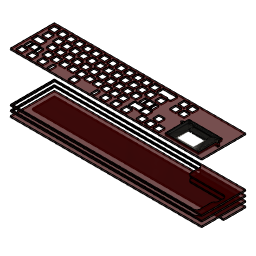
Snack  Case Concept V1 v1 (Autodesk Fusion 360 design; units mm, degrees)
Autodesk Fusion 360 part; units mm, degrees
(part 1 of 3)
sketch "plate-20210524-013526" plane through (0, 0, 0) normal (0, 0, 1) x (1, 0, 0)
  line L0 (286.3938, -78.725) -> (299.3938, -78.725)
  arc A0 (285.8938, -92.225) -> (286.3938, -92.725) centre (286.3938, -92.225) ccw
  arc A1 (299.3938, -92.725) -> (299.8938, -92.225) centre (299.3938, -92.225) ccw
  arc A2 (373.7125, -79.225) -> (373.2125, -78.725) centre (373.2125, -79.225) ccw
  arc A3 (359.7125, -92.225) -> (360.2125, -92.725) centre (360.2125, -92.225) ccw
  arc A4 (276.0813, -79.225) -> (275.5813, -78.725) centre (275.5813, -79.225) ccw
  arc A5 (354.6625, -79.225) -> (354.1625, -78.725) centre (354.1625, -79.225) ccw
  arc A6 (354.1625, -92.725) -> (354.6625, -92.225) centre (354.1625, -92.225) ccw
  line L1 (341.1625, -78.725) -> (354.1625, -78.725)
  arc A7 (335.1125, -92.725) -> (335.6125, -92.225) centre (335.1125, -92.225) ccw
  arc A8 (335.6125, -79.225) -> (335.1125, -78.725) centre (335.1125, -79.225) ccw
  arc A9 (340.6625, -92.225) -> (341.1625, -92.725) centre (341.1625, -92.225) ccw
  line L2 (360.2125, -92.725) -> (373.2125, -92.725)
  line L3 (373.7125, -79.225) -> (373.7125, -92.225)
  line L4 (299.8938, -79.225) -> (299.8938, -92.225)
  line L5 (322.1125, -78.725) -> (335.1125, -78.725)
  arc A10 (321.6125, -92.225) -> (322.1125, -92.725) centre (322.1125, -92.225) ccw
  line L6 (354.6625, -79.225) -> (354.6625, -92.225)
  line L7 (285.8938, -79.225) -> (285.8938, -92.225)
  line L8 (359.7125, -79.225) -> (359.7125, -92.225)
  line L9 (322.1125, -92.725) -> (335.1125, -92.725)
  line L10 (286.3938, -92.725) -> (299.3938, -92.725)
  line L11 (341.1625, -92.725) -> (354.1625, -92.725)
  line L12 (360.2125, -78.725) -> (373.2125, -78.725)
  arc A11 (322.1125, -78.725) -> (321.6125, -79.225) centre (322.1125, -79.225) ccw
  arc A12 (341.1625, -78.725) -> (340.6625, -79.225) centre (341.1625, -79.225) ccw
  line L13 (335.6125, -79.225) -> (335.6125, -92.225)
  arc A13 (286.3938, -78.725) -> (285.8938, -79.225) centre (286.3938, -79.225) ccw
  arc A14 (275.5813, -92.725) -> (276.0813, -92.225) centre (275.5813, -92.225) ccw
  arc A15 (360.2125, -78.725) -> (359.7125, -79.225) centre (360.2125, -79.225) ccw
  arc A16 (45.3875, -16.025) -> (45.8875, -16.525) centre (45.8875, -16.025) ccw
  arc A17 (299.8938, -79.225) -> (299.3938, -78.725) centre (299.3938, -79.225) ccw
  arc A18 (262.0813, -92.225) -> (262.5813, -92.725) centre (262.5813, -92.225) ccw
  line L14 (321.6125, -79.225) -> (321.6125, -92.225)
  line L15 (340.6625, -79.225) -> (340.6625, -92.225)
  arc A19 (373.2125, -92.725) -> (373.7125, -92.225) centre (373.2125, -92.225) ccw
  line L16 (64.4375, -3.025) -> (64.4375, -16.025)
  line L17 (160.1875, -2.525) -> (173.1875, -2.525)
  line L18 (135.5875, -3.025) -> (135.5875, -16.025)
  arc A20 (116.5375, -3.025) -> (116.0375, -2.525) centre (116.0375, -3.025) ccw
  arc A21 (58.8875, -16.525) -> (59.3875, -16.025) centre (58.8875, -16.025) ccw
  arc A22 (160.1875, -2.525) -> (159.6875, -3.025) centre (160.1875, -3.025) ccw
  arc A23 (173.1875, -16.525) -> (173.6875, -16.025) centre (173.1875, -16.025) ccw
  arc A24 (97.4875, -3.025) -> (96.9875, -2.525) centre (96.9875, -3.025) ccw
  line L19 (140.6375, -3.025) -> (140.6375, -16.025)
  line L20 (178.7375, -3.025) -> (178.7375, -16.025)
  arc A25 (83.4875, -16.025) -> (83.9875, -16.525) centre (83.9875, -16.025) ccw
  line L21 (160.1875, -16.525) -> (173.1875, -16.525)
  arc A26 (159.6875, -16.025) -> (160.1875, -16.525) centre (160.1875, -16.025) ccw
  arc A27 (64.4375, -16.025) -> (64.9375, -16.525) centre (64.9375, -16.025) ccw
  arc A28 (45.8875, -2.525) -> (45.3875, -3.025) centre (45.8875, -3.025) ccw
  arc A29 (102.5375, -16.025) -> (103.0375, -16.525) centre (103.0375, -16.025) ccw
  line L22 (78.4375, -3.025) -> (78.4375, -16.025)
  arc A30 (154.6375, -3.025) -> (154.1375, -2.525) centre (154.1375, -3.025) ccw
  arc A31 (135.0875, -16.525) -> (135.5875, -16.025) centre (135.0875, -16.025) ccw
  line L23 (64.9375, -2.525) -> (77.9375, -2.525)
  line L24 (141.1375, -2.525) -> (154.1375, -2.525)
  line L25 (121.5875, -3.025) -> (121.5875, -16.025)
  line L26 (154.6375, -3.025) -> (154.6375, -16.025)
  line L27 (102.5375, -3.025) -> (102.5375, -16.025)
  line L28 (159.6875, -3.025) -> (159.6875, -16.025)
  line L29 (45.3875, -3.025) -> (45.3875, -16.025)
  line L30 (122.0875, -2.525) -> (135.0875, -2.525)
  arc A32 (116.0375, -16.525) -> (116.5375, -16.025) centre (116.0375, -16.025) ccw
  line L31 (103.0375, -2.525) -> (116.0375, -2.525)
  line L32 (179.2375, -16.525) -> (192.2375, -16.525)
  line L33 (83.4875, -3.025) -> (83.4875, -16.025)
  line L34 (116.5375, -3.025) -> (116.5375, -16.025)
  line L35 (103.0375, -16.525) -> (116.0375, -16.525)
  line L36 (97.4875, -3.025) -> (97.4875, -16.025)
  arc A33 (59.3875, -3.025) -> (58.8875, -2.525) centre (58.8875, -3.025) ccw
  line L37 (192.7375, -3.025) -> (192.7375, -16.025)
  arc A34 (141.1375, -2.525) -> (140.6375, -3.025) centre (141.1375, -3.025) ccw
  arc A35 (64.9375, -2.525) -> (64.4375, -3.025) centre (64.9375, -3.025) ccw
  arc A36 (77.9375, -16.525) -> (78.4375, -16.025) centre (77.9375, -16.025) ccw
  arc A37 (135.5875, -3.025) -> (135.0875, -2.525) centre (135.0875, -3.025) ccw
  line L38 (64.9375, -16.525) -> (77.9375, -16.525)
  arc A38 (122.0875, -2.525) -> (121.5875, -3.025) centre (122.0875, -3.025) ccw
  arc A39 (268.9375, -3.025) -> (268.4375, -2.525) centre (268.4375, -3.025) ccw
  arc A40 (198.2875, -2.525) -> (197.7875, -3.025) centre (198.2875, -3.025) ccw
  line L39 (235.8875, -3.025) -> (235.8875, -16.025)
  line L40 (236.3875, -2.525) -> (249.3875, -2.525)
  arc A41 (287.9875, -3.025) -> (287.4875, -2.525) centre (287.4875, -3.025) ccw
  arc A42 (274.4875, -2.525) -> (273.9875, -3.025) centre (274.4875, -3.025) ccw
  arc A43 (236.3875, -2.525) -> (235.8875, -3.025) centre (236.3875, -3.025) ccw
  line L41 (294.1245, -17.025) -> (294.1245, -18.025)
  arc A44 (121.5875, -16.025) -> (122.0875, -16.525) centre (122.0875, -16.025) ccw
  arc A45 (83.9875, -2.525) -> (83.4875, -3.025) centre (83.9875, -3.025) ccw
  line L42 (83.9875, -16.525) -> (96.9875, -16.525)
  line L43 (122.0875, -16.525) -> (135.0875, -16.525)
  line L44 (198.2875, -2.525) -> (211.2875, -2.525)
  line L45 (83.9875, -2.525) -> (96.9875, -2.525)
  arc A46 (324.5005, -18.525) -> (325.0005, -18.025) centre (324.5005, -18.025) ccw
  line L46 (294.6245, -18.525) -> (300.6245, -18.525)
  arc A47 (178.7375, -16.025) -> (179.2375, -16.525) centre (179.2375, -16.025) ccw
  line L47 (301.1245, -17.025) -> (301.1245, -18.025)
  line L48 (254.9375, -3.025) -> (254.9375, -16.025)
  arc A48 (230.8375, -3.025) -> (230.3375, -2.525) centre (230.3375, -3.025) ccw
  line L49 (230.8375, -3.025) -> (230.8375, -16.025)
  line L50 (45.8875, -2.525) -> (58.8875, -2.525)
  line L51 (273.9875, -3.025) -> (273.9875, -16.025)
  line L52 (141.1375, -16.525) -> (154.1375, -16.525)
  line L53 (197.7875, -3.025) -> (197.7875, -16.025)
  arc A49 (249.8875, -3.025) -> (249.3875, -2.525) centre (249.3875, -3.025) ccw
  line L54 (216.8375, -3.025) -> (216.8375, -16.025)
  line L55 (249.8875, -3.025) -> (249.8875, -16.025)
  arc A50 (217.3375, -2.525) -> (216.8375, -3.025) centre (217.3375, -3.025) ccw
  arc A51 (216.8375, -16.025) -> (217.3375, -16.525) centre (217.3375, -16.025) ccw
  line L56 (268.9375, -3.025) -> (268.9375, -16.025)
  line L57 (45.8875, -16.525) -> (58.8875, -16.525)
  arc A52 (140.6375, -16.025) -> (141.1375, -16.525) centre (141.1375, -16.025) ccw
  line L58 (179.2375, -2.525) -> (192.2375, -2.525)
  line L59 (217.3375, -16.525) -> (230.3375, -16.525)
  arc A53 (197.7875, -16.025) -> (198.2875, -16.525) centre (198.2875, -16.025) ccw
  arc A54 (273.9875, -16.025) -> (274.4875, -16.525) centre (274.4875, -16.025) ccw
  arc A55 (96.9875, -16.525) -> (97.4875, -16.025) centre (96.9875, -16.025) ccw
  line L60 (236.3875, -16.525) -> (249.3875, -16.525)
  line L61 (59.3875, -3.025) -> (59.3875, -16.025)
  line L62 (303.0625, -2.525) -> (316.0625, -2.525)
  arc A56 (235.8875, -16.025) -> (236.3875, -16.525) centre (236.3875, -16.025) ccw
  arc A57 (268.4375, -16.525) -> (268.9375, -16.025) centre (268.4375, -16.025) ccw
  arc A58 (211.2875, -16.525) -> (211.7875, -16.025) centre (211.2875, -16.025) ccw
  line L63 (173.6875, -3.025) -> (173.6875, -16.025)
  line L64 (318.5005, -18.525) -> (324.5005, -18.525)
  line L65 (211.7875, -3.025) -> (211.7875, -16.025)
  arc A59 (78.4375, -3.025) -> (77.9375, -2.525) centre (77.9375, -3.025) ccw
  arc A60 (103.0375, -2.525) -> (102.5375, -3.025) centre (103.0375, -3.025) ccw
  arc A61 (255.4375, -2.525) -> (254.9375, -3.025) centre (255.4375, -3.025) ccw
  line L66 (255.4375, -2.525) -> (268.4375, -2.525)
  arc A62 (154.1375, -16.525) -> (154.6375, -16.025) centre (154.1375, -16.025) ccw
  arc A63 (173.6875, -3.025) -> (173.1875, -2.525) centre (173.1875, -3.025) ccw
  arc A64 (192.7375, -3.025) -> (192.2375, -2.525) centre (192.2375, -3.025) ccw
  arc A65 (179.2375, -2.525) -> (178.7375, -3.025) centre (179.2375, -3.025) ccw
  arc A66 (211.7875, -3.025) -> (211.2875, -2.525) centre (211.2875, -3.025) ccw
  line L67 (255.4375, -16.525) -> (268.4375, -16.525)
  line L68 (274.4875, -16.525) -> (287.4875, -16.525)
  line L69 (131.1125, -22.075) -> (131.1125, -35.075)
  line L70 (74.4625, -21.575) -> (87.4625, -21.575)
  line L71 (287.9875, -3.025) -> (287.9875, -16.025)
  arc A67 (287.4875, -16.525) -> (287.9875, -16.025) centre (287.4875, -16.025) ccw
  arc A68 (318.0005, -18.025) -> (318.5005, -18.525) centre (318.5005, -18.025) ccw
  arc A69 (64.15, -22.075) -> (63.65, -21.575) centre (63.65, -22.075) ccw
  arc A70 (126.0625, -22.075) -> (125.5625, -21.575) centre (125.5625, -22.075) ccw
  line L72 (131.6125, -35.575) -> (144.6125, -35.575)
  line L73 (50.65, -35.575) -> (63.65, -35.575)
  line L74 (73.9625, -22.075) -> (73.9625, -35.075)
  arc A71 (373.2125, -16.525) -> (373.7125, -16.025) centre (373.2125, -16.025) ccw
  arc A72 (300.6245, -18.525) -> (301.1245, -18.025) centre (300.6245, -18.025) ccw
  line L75 (217.3375, -2.525) -> (230.3375, -2.525)
  arc A73 (144.6125, -35.575) -> (145.1125, -35.075) centre (144.6125, -35.075) ccw
  arc A74 (192.2375, -16.525) -> (192.7375, -16.025) centre (192.2375, -16.025) ccw
  line L76 (126.0625, -22.075) -> (126.0625, -35.075)
  arc A75 (50.65, -21.575) -> (50.15, -22.075) centre (50.65, -22.075) ccw
  line L77 (150.6625, -35.575) -> (163.6625, -35.575)
  arc A76 (93.5125, -21.575) -> (93.0125, -22.075) centre (93.5125, -22.075) ccw
  arc A77 (230.3375, -16.525) -> (230.8375, -16.025) centre (230.3375, -16.025) ccw
  line L78 (198.2875, -16.525) -> (211.2875, -16.525)
  arc A78 (87.9625, -22.075) -> (87.4625, -21.575) centre (87.4625, -22.075) ccw
  line L79 (107.0125, -22.075) -> (107.0125, -35.075)
  line L80 (373.7125, -3.025) -> (373.7125, -16.025)
  line L81 (150.1625, -22.075) -> (150.1625, -35.075)
  arc A79 (254.9375, -16.025) -> (255.4375, -16.525) centre (255.4375, -16.025) ccw
  arc A80 (360.2125, -2.525) -> (359.7125, -3.025) centre (360.2125, -3.025) ccw
  line L82 (325.0005, -17.025) -> (325.0005, -18.025)
  line L83 (354.6625, -3.025) -> (354.6625, -16.025)
  arc A81 (145.1125, -22.075) -> (144.6125, -21.575) centre (144.6125, -22.075) ccw
  line L84 (164.1625, -22.075) -> (164.1625, -35.075)
  line L85 (341.1625, -16.525) -> (354.1625, -16.525)
  arc A82 (107.0125, -22.075) -> (106.5125, -21.575) centre (106.5125, -22.075) ccw
  arc A83 (87.4625, -35.575) -> (87.9625, -35.075) centre (87.4625, -35.075) ccw
  line L86 (93.5125, -35.575) -> (106.5125, -35.575)
  arc A84 (73.9625, -35.075) -> (74.4625, -35.575) centre (74.4625, -35.075) ccw
  arc A85 (354.1625, -16.525) -> (354.6625, -16.025) centre (354.1625, -16.025) ccw
  line L87 (93.0125, -22.075) -> (93.0125, -35.075)
  line L88 (274.4875, -2.525) -> (287.4875, -2.525)
  arc A86 (373.7125, -3.025) -> (373.2125, -2.525) centre (373.2125, -3.025) ccw
  arc A87 (50.15, -35.075) -> (50.65, -35.575) centre (50.65, -35.075) ccw
  line L89 (112.5625, -21.575) -> (125.5625, -21.575)
  line L90 (360.2125, -2.525) -> (373.2125, -2.525)
  arc A88 (93.0125, -35.075) -> (93.5125, -35.575) centre (93.5125, -35.075) ccw
  line L91 (150.6625, -21.575) -> (163.6625, -21.575)
  arc A89 (74.4625, -21.575) -> (73.9625, -22.075) centre (74.4625, -22.075) ccw
  line L92 (360.2125, -16.525) -> (373.2125, -16.525)
  line L93 (64.15, -22.075) -> (64.15, -35.075)
  arc A90 (112.0625, -35.075) -> (112.5625, -35.575) centre (112.5625, -35.075) ccw
  arc A91 (340.6625, -16.025) -> (341.1625, -16.525) centre (341.1625, -16.025) ccw
  arc A92 (249.3875, -16.525) -> (249.8875, -16.025) centre (249.3875, -16.025) ccw
  line L94 (145.1125, -22.075) -> (145.1125, -35.075)
  line L95 (318.0005, -17.025) -> (318.0005, -18.025)
  arc A93 (125.5625, -35.575) -> (126.0625, -35.075) centre (125.5625, -35.075) ccw
  line L96 (303.0625, -16.525) -> (316.0625, -16.525)
  arc A94 (354.6625, -3.025) -> (354.1625, -2.525) centre (354.1625, -3.025) ccw
  line L97 (87.9625, -22.075) -> (87.9625, -35.075)
  arc A95 (131.6125, -21.575) -> (131.1125, -22.075) centre (131.6125, -22.075) ccw
  line L98 (50.15, -22.075) -> (50.15, -35.075)
  line L99 (359.7125, -3.025) -> (359.7125, -16.025)
  arc A96 (245.4125, -35.075) -> (245.9125, -35.575) centre (245.9125, -35.075) ccw
  line L100 (183.2125, -22.075) -> (183.2125, -35.075)
  line L101 (278.4625, -22.075) -> (278.4625, -35.075)
  line L102 (226.8625, -35.575) -> (239.8625, -35.575)
  arc A97 (131.1125, -35.075) -> (131.6125, -35.575) centre (131.6125, -35.075) ccw
  line L103 (341.1625, -2.525) -> (354.1625, -2.525)
  arc A98 (226.3625, -35.075) -> (226.8625, -35.575) centre (226.8625, -35.075) ccw
  line L104 (283.5125, -22.075) -> (283.5125, -35.075)
  line L105 (188.2625, -22.075) -> (188.2625, -35.075)
  arc A99 (182.7125, -35.575) -> (183.2125, -35.075) centre (182.7125, -35.075) ccw
  line L106 (74.4625, -35.575) -> (87.4625, -35.575)
  arc A100 (220.8125, -35.575) -> (221.3125, -35.075) centre (220.8125, -35.075) ccw
  line L107 (307.825, -21.575) -> (320.825, -21.575)
  arc A101 (221.3125, -22.075) -> (220.8125, -21.575) centre (220.8125, -22.075) ccw
  line L108 (188.7625, -35.575) -> (201.7625, -35.575)
  arc A102 (258.9125, -35.575) -> (259.4125, -35.075) centre (258.9125, -35.075) ccw
  line L109 (340.6625, -3.025) -> (340.6625, -16.025)
  line L110 (169.7125, -35.575) -> (182.7125, -35.575)
  line L111 (240.3625, -22.075) -> (240.3625, -35.075)
  line L112 (221.3125, -22.075) -> (221.3125, -35.075)
  arc A103 (202.2625, -22.075) -> (201.7625, -21.575) centre (201.7625, -22.075) ccw
  line L113 (264.9625, -21.575) -> (277.9625, -21.575)
  line L114 (226.3625, -22.075) -> (226.3625, -35.075)
  line L115 (93.5125, -21.575) -> (106.5125, -21.575)
  line L116 (188.7625, -21.575) -> (201.7625, -21.575)
  line L117 (169.2125, -22.075) -> (169.2125, -35.075)
  line L118 (226.8625, -21.575) -> (239.8625, -21.575)
  line L119 (112.5625, -35.575) -> (125.5625, -35.575)
  line L120 (245.9125, -35.575) -> (258.9125, -35.575)
  line L121 (131.6125, -21.575) -> (144.6125, -21.575)
  arc A104 (240.3625, -22.075) -> (239.8625, -21.575) centre (239.8625, -22.075) ccw
  arc A105 (264.9625, -21.575) -> (264.4625, -22.075) centre (264.9625, -22.075) ccw
  line L122 (284.0125, -35.575) -> (297.0125, -35.575)
  arc A106 (163.6625, -35.575) -> (164.1625, -35.075) centre (163.6625, -35.075) ccw
  arc A107 (359.7125, -16.025) -> (360.2125, -16.525) centre (360.2125, -16.025) ccw
  arc A108 (106.5125, -35.575) -> (107.0125, -35.075) centre (106.5125, -35.075) ccw
  arc A109 (278.4625, -22.075) -> (277.9625, -21.575) centre (277.9625, -22.075) ccw
  line L123 (259.4125, -22.075) -> (259.4125, -35.075)
  line L124 (207.8125, -35.575) -> (220.8125, -35.575)
  arc A110 (277.9625, -35.575) -> (278.4625, -35.075) centre (277.9625, -35.075) ccw
  arc A111 (259.4125, -22.075) -> (258.9125, -21.575) centre (258.9125, -22.075) ccw
  arc A112 (284.0125, -21.575) -> (283.5125, -22.075) centre (284.0125, -22.075) ccw
  line L125 (50.65, -21.575) -> (63.65, -21.575)
  arc A113 (63.65, -35.575) -> (64.15, -35.075) centre (63.65, -35.075) ccw
  line L126 (321.325, -22.075) -> (321.325, -35.075)
  arc A114 (188.7625, -21.575) -> (188.2625, -22.075) centre (188.7625, -22.075) ccw
  line L127 (284.0125, -21.575) -> (297.0125, -21.575)
  line L128 (297.5125, -22.075) -> (297.5125, -35.075)
  arc A115 (169.7125, -21.575) -> (169.2125, -22.075) centre (169.7125, -22.075) ccw
  arc A116 (283.5125, -35.075) -> (284.0125, -35.575) centre (284.0125, -35.075) ccw
  line L129 (264.4625, -22.075) -> (264.4625, -35.075)
  line L130 (307.825, -35.575) -> (320.825, -35.575)
  arc A117 (112.5625, -21.575) -> (112.0625, -22.075) centre (112.5625, -22.075) ccw
  arc A118 (245.9125, -21.575) -> (245.4125, -22.075) centre (245.9125, -22.075) ccw
  arc A119 (164.1625, -22.075) -> (163.6625, -21.575) centre (163.6625, -22.075) ccw
  arc A120 (341.1625, -2.525) -> (340.6625, -3.025) centre (341.1625, -3.025) ccw
  arc A121 (239.8625, -35.575) -> (240.3625, -35.075) centre (239.8625, -35.075) ccw
  arc A122 (294.1245, -18.025) -> (294.6245, -18.525) centre (294.6245, -18.025) ccw
  arc A123 (183.2125, -22.075) -> (182.7125, -21.575) centre (182.7125, -22.075) ccw
  line L131 (112.0625, -22.075) -> (112.0625, -35.075)
  arc A124 (264.4625, -35.075) -> (264.9625, -35.575) centre (264.9625, -35.075) ccw
  line L132 (66.5312, -41.125) -> (66.5312, -54.125)
  arc A125 (150.1625, -35.075) -> (150.6625, -35.575) centre (150.6625, -35.075) ccw
  arc A126 (354.6625, -22.075) -> (354.1625, -21.575) centre (354.1625, -22.075) ccw
  line L133 (202.2625, -22.075) -> (202.2625, -35.075)
  arc A127 (360.2125, -21.575) -> (359.7125, -22.075) centre (360.2125, -22.075) ccw
  arc A128 (307.825, -21.575) -> (307.325, -22.075) centre (307.825, -22.075) ccw
  line L134 (207.3125, -22.075) -> (207.3125, -35.075)
  line L135 (245.9125, -21.575) -> (258.9125, -21.575)
  line L136 (117.325, -40.625) -> (130.325, -40.625)
  line L137 (53.0313, -54.625) -> (66.0312, -54.625)
  arc A129 (116.825, -54.125) -> (117.325, -54.625) centre (117.325, -54.125) ccw
  line L138 (79.225, -40.625) -> (92.225, -40.625)
  arc A130 (78.725, -54.125) -> (79.225, -54.625) centre (79.225, -54.125) ccw
  line L139 (360.2125, -21.575) -> (373.2125, -21.575)
  line L140 (92.725, -41.125) -> (92.725, -54.125)
  arc A131 (45.3875, -54.125) -> (45.8875, -54.625) centre (45.8875, -54.125) ccw
  arc A132 (207.3125, -35.075) -> (207.8125, -35.575) centre (207.8125, -35.075) ccw
  arc A133 (188.2625, -35.075) -> (188.7625, -35.575) centre (188.7625, -35.075) ccw
  arc A134 (207.8125, -21.575) -> (207.3125, -22.075) centre (207.8125, -22.075) ccw
  line L141 (136.375, -40.625) -> (149.375, -40.625)
  line L142 (341.1625, -35.575) -> (354.1625, -35.575)
  arc A135 (373.7125, -22.075) -> (373.2125, -21.575) centre (373.2125, -22.075) ccw
  arc A136 (98.275, -40.625) -> (97.775, -41.125) centre (98.275, -41.125) ccw
  arc A137 (130.325, -54.625) -> (130.825, -54.125) centre (130.325, -54.125) ccw
  line L143 (169.7125, -21.575) -> (182.7125, -21.575)
  arc A138 (297.0125, -35.575) -> (297.5125, -35.075) centre (297.0125, -35.075) ccw
  arc A139 (201.7625, -35.575) -> (202.2625, -35.075) centre (201.7625, -35.075) ccw
  arc A140 (97.775, -54.125) -> (98.275, -54.625) centre (98.275, -54.125) ccw
  line L144 (78.725, -41.125) -> (78.725, -54.125)
  arc A141 (354.1625, -35.575) -> (354.6625, -35.075) centre (354.1625, -35.075) ccw
  line L145 (98.275, -54.625) -> (111.275, -54.625)
  line L146 (245.4125, -22.075) -> (245.4125, -35.075)
  arc A142 (130.825, -41.125) -> (130.325, -40.625) centre (130.325, -41.125) ccw
  arc A143 (92.725, -41.125) -> (92.225, -40.625) centre (92.225, -41.125) ccw
  line L147 (130.825, -41.125) -> (130.825, -54.125)
  line L148 (79.225, -54.625) -> (92.225, -54.625)
  arc A144 (297.5125, -22.075) -> (297.0125, -21.575) centre (297.0125, -22.075) ccw
  line L149 (97.775, -41.125) -> (97.775, -54.125)
  arc A145 (169.2125, -35.075) -> (169.7125, -35.575) centre (169.7125, -35.075) ccw
  line L150 (307.325, -22.075) -> (307.325, -35.075)
  arc A146 (150.6625, -21.575) -> (150.1625, -22.075) centre (150.6625, -22.075) ccw
  arc A147 (111.275, -54.625) -> (111.775, -54.125) centre (111.275, -54.125) ccw
  line L151 (116.825, -41.125) -> (116.825, -54.125)
  arc A148 (117.325, -40.625) -> (116.825, -41.125) centre (117.325, -41.125) ccw
  line L152 (207.8125, -21.575) -> (220.8125, -21.575)
  line L153 (117.325, -54.625) -> (130.325, -54.625)
  arc A149 (45.8875, -40.625) -> (45.3875, -41.125) centre (45.8875, -41.125) ccw
  line L154 (341.1625, -21.575) -> (354.1625, -21.575)
  line L155 (340.6625, -22.075) -> (340.6625, -35.075)
  line L156 (373.7125, -22.075) -> (373.7125, -35.075)
  arc A150 (340.6625, -35.075) -> (341.1625, -35.575) centre (341.1625, -35.075) ccw
  line L157 (360.2125, -35.575) -> (373.2125, -35.575)
  line L158 (354.6625, -22.075) -> (354.6625, -35.075)
  arc A151 (226.8625, -21.575) -> (226.3625, -22.075) centre (226.8625, -22.075) ccw
  arc A152 (92.225, -54.625) -> (92.725, -54.125) centre (92.225, -54.125) ccw
  arc A153 (111.775, -41.125) -> (111.275, -40.625) centre (111.275, -41.125) ccw
  arc A154 (66.5312, -41.125) -> (66.0312, -40.625) centre (66.0312, -41.125) ccw
  arc A155 (320.825, -35.575) -> (321.325, -35.075) centre (320.825, -35.075) ccw
  arc A156 (66.0312, -54.625) -> (66.5312, -54.125) centre (66.0312, -54.125) ccw
  line L159 (264.9625, -35.575) -> (277.9625, -35.575)
  line L160 (212.075, -41.125) -> (212.075, -54.125)
  arc A157 (136.375, -40.625) -> (135.875, -41.125) centre (136.375, -41.125) ccw
  line L161 (245.125, -41.125) -> (245.125, -54.125)
  arc A158 (231.625, -40.625) -> (231.125, -41.125) centre (231.625, -41.125) ccw
  line L162 (98.275, -40.625) -> (111.275, -40.625)
  arc A159 (341.1625, -21.575) -> (340.6625, -22.075) centre (341.1625, -22.075) ccw
  arc A160 (264.175, -41.125) -> (263.675, -40.625) centre (263.675, -41.125) ccw
  line L163 (300.6812, -54.625) -> (313.6812, -54.625)
  line L164 (250.675, -40.625) -> (263.675, -40.625)
  arc A161 (193.525, -40.625) -> (193.025, -41.125) centre (193.525, -41.125) ccw
  arc A162 (154.925, -54.125) -> (155.425, -54.625) centre (155.425, -54.125) ccw
  arc A163 (187.475, -54.625) -> (187.975, -54.125) centre (187.475, -54.125) ccw
  line L165 (212.575, -40.625) -> (225.575, -40.625)
  line L166 (174.475, -40.625) -> (187.475, -40.625)
  arc A164 (193.025, -54.125) -> (193.525, -54.625) centre (193.525, -54.125) ccw
  arc A165 (321.325, -22.075) -> (320.825, -21.575) centre (320.825, -22.075) ccw
  line L167 (149.875, -41.125) -> (149.875, -54.125)
  arc A166 (79.225, -40.625) -> (78.725, -41.125) centre (79.225, -41.125) ccw
  line L168 (359.7125, -22.075) -> (359.7125, -35.075)
  arc A167 (283.225, -41.125) -> (282.725, -40.625) centre (282.725, -41.125) ccw
  line L169 (136.375, -54.625) -> (149.375, -54.625)
  line L170 (300.6812, -40.625) -> (313.6812, -40.625)
  line L171 (187.975, -41.125) -> (187.975, -54.125)
  arc A168 (226.075, -41.125) -> (225.575, -40.625) centre (225.575, -41.125) ccw
  line L172 (250.675, -54.625) -> (263.675, -54.625)
  arc A169 (307.325, -35.075) -> (307.825, -35.575) centre (307.825, -35.075) ccw
  line L173 (264.175, -41.125) -> (264.175, -54.125)
  arc A170 (212.075, -54.125) -> (212.575, -54.625) centre (212.575, -54.125) ccw
  line L174 (154.925, -41.125) -> (154.925, -54.125)
  arc A171 (269.225, -54.125) -> (269.725, -54.625) centre (269.725, -54.125) ccw
  line L175 (174.475, -54.625) -> (187.475, -54.625)
  line L176 (45.3875, -41.125) -> (45.3875, -54.125)
  line L177 (231.625, -54.625) -> (244.625, -54.625)
  arc A172 (359.7125, -35.075) -> (360.2125, -35.575) centre (360.2125, -35.075) ccw
  line L178 (269.225, -41.125) -> (269.225, -54.125)
  line L179 (135.875, -41.125) -> (135.875, -54.125)
  arc A173 (373.2125, -35.575) -> (373.7125, -35.075) centre (373.2125, -35.075) ccw
  arc A174 (282.725, -54.625) -> (283.225, -54.125) centre (282.725, -54.125) ccw
  line L180 (300.1812, -41.125) -> (300.1812, -54.125)
  line L181 (193.025, -41.125) -> (193.025, -54.125)
  arc A175 (168.425, -54.625) -> (168.925, -54.125) centre (168.425, -54.125) ccw
  arc A176 (207.025, -41.125) -> (206.525, -40.625) centre (206.525, -41.125) ccw
  line L182 (111.775, -41.125) -> (111.775, -54.125)
  line L183 (53.0313, -40.625) -> (66.0312, -40.625)
  arc A177 (187.975, -41.125) -> (187.475, -40.625) centre (187.475, -41.125) ccw
  line L184 (155.425, -40.625) -> (168.425, -40.625)
  line L185 (269.725, -40.625) -> (282.725, -40.625)
  line L186 (207.025, -41.125) -> (207.025, -54.125)
  line L187 (45.8875, -54.625) -> (58.8875, -54.625)
  arc A178 (168.925, -41.125) -> (168.425, -40.625) centre (168.425, -41.125) ccw
  arc A179 (149.875, -41.125) -> (149.375, -40.625) centre (149.375, -41.125) ccw
  line L188 (168.925, -41.125) -> (168.925, -54.125)
  line L189 (269.725, -54.625) -> (282.725, -54.625)
  line L190 (173.975, -41.125) -> (173.975, -54.125)
  line L191 (45.8875, -40.625) -> (58.8875, -40.625)
  line L192 (314.1812, -41.125) -> (314.1812, -54.125)
  arc A180 (155.425, -40.625) -> (154.925, -41.125) centre (155.425, -41.125) ccw
  line L193 (193.525, -40.625) -> (206.525, -40.625)
  arc A181 (149.375, -54.625) -> (149.875, -54.125) centre (149.375, -54.125) ccw
  arc A182 (212.575, -40.625) -> (212.075, -41.125) centre (212.575, -41.125) ccw
  arc A183 (231.125, -54.125) -> (231.625, -54.625) centre (231.625, -54.125) ccw
  line L194 (231.625, -40.625) -> (244.625, -40.625)
  line L195 (57.7938, -59.675) -> (70.7938, -59.675)
  line L196 (193.525, -54.625) -> (206.525, -54.625)
  line L197 (73.2318, -75.675) -> (79.2318, -75.675)
  line L198 (107.8, -73.675) -> (120.8, -73.675)
  arc A184 (72.7318, -75.175) -> (73.2318, -75.675) centre (73.2318, -75.175) ccw
  arc A185 (244.625, -54.625) -> (245.125, -54.125) centre (244.625, -54.125) ccw
  line L199 (155.425, -54.625) -> (168.425, -54.625)
  line L200 (315.6193, -42.125) -> (315.6193, -56.125)
  arc A186 (70.7938, -73.675) -> (71.2938, -73.175) centre (70.7938, -73.175) ccw
  arc A187 (292.2432, -41.625) -> (291.7432, -42.125) centre (292.2432, -42.125) ccw
  arc A188 (73.2318, -60.675) -> (72.7318, -61.175) centre (73.2318, -61.175) ccw
  line L201 (298.7432, -42.125) -> (298.7432, -56.125)
  line L202 (121.3, -60.175) -> (121.3, -73.175)
  line L203 (226.075, -41.125) -> (226.075, -54.125)
  arc A189 (120.8, -73.675) -> (121.3, -73.175) centre (120.8, -73.175) ccw
  arc A190 (48.8558, -75.175) -> (49.3558, -75.675) centre (49.3558, -75.175) ccw
  line L204 (57.2938, -60.175) -> (57.2938, -73.175)
  line L205 (316.1193, -41.625) -> (322.1193, -41.625)
  line L206 (49.3558, -75.675) -> (55.3558, -75.675)
  arc A191 (206.525, -54.625) -> (207.025, -54.125) centre (206.525, -54.125) ccw
  arc A192 (313.6812, -54.625) -> (314.1812, -54.125) centre (313.6812, -54.125) ccw
  line L207 (126.85, -59.675) -> (139.85, -59.675)
  line L208 (55.8558, -61.175) -> (55.8558, -75.175)
  line L209 (283.225, -41.125) -> (283.225, -54.125)
  arc A193 (173.975, -54.125) -> (174.475, -54.625) centre (174.475, -54.125) ccw
  line L210 (57.7938, -73.675) -> (70.7938, -73.675)
  arc A194 (245.125, -41.125) -> (244.625, -40.625) centre (244.625, -41.125) ccw
  line L211 (126.85, -73.675) -> (139.85, -73.675)
  arc A195 (300.1812, -54.125) -> (300.6812, -54.625) centre (300.6812, -54.125) ccw
  arc A196 (135.875, -54.125) -> (136.375, -54.625) centre (136.375, -54.125) ccw
  arc A197 (102.25, -60.175) -> (101.75, -59.675) centre (101.75, -60.175) ccw
  arc A198 (55.8558, -61.175) -> (55.3558, -60.675) centre (55.3558, -61.175) ccw
  line L212 (102.25, -60.175) -> (102.25, -73.175)
  line L213 (140.35, -60.175) -> (140.35, -73.175)
  line L214 (231.125, -41.125) -> (231.125, -54.125)
  arc A199 (263.675, -54.625) -> (264.175, -54.125) centre (263.675, -54.125) ccw
  arc A200 (57.2938, -73.175) -> (57.7938, -73.675) centre (57.7938, -73.175) ccw
  line L215 (292.2432, -56.625) -> (298.2432, -56.625)
  arc A201 (291.7432, -56.125) -> (292.2432, -56.625) centre (292.2432, -56.125) ccw
  arc A202 (71.2938, -60.175) -> (70.7938, -59.675) centre (70.7938, -60.175) ccw
  arc A203 (225.575, -54.625) -> (226.075, -54.125) centre (225.575, -54.125) ccw
  arc A204 (107.8, -59.675) -> (107.3, -60.175) centre (107.8, -60.175) ccw
  arc A205 (250.675, -40.625) -> (250.175, -41.125) centre (250.675, -41.125) ccw
  arc A206 (250.175, -54.125) -> (250.675, -54.625) centre (250.675, -54.125) ccw
  line L216 (212.575, -54.625) -> (225.575, -54.625)
  line L217 (250.175, -41.125) -> (250.175, -54.125)
  arc A207 (107.3, -73.175) -> (107.8, -73.675) centre (107.8, -73.175) ccw
  arc A208 (314.1812, -41.125) -> (313.6812, -40.625) centre (313.6812, -41.125) ccw
  line L218 (126.35, -60.175) -> (126.35, -73.175)
  line L219 (79.7318, -61.175) -> (79.7318, -75.175)
  arc A209 (322.6192, -42.125) -> (322.1193, -41.625) centre (322.1193, -42.125) ccw
  arc A210 (121.3, -60.175) -> (120.8, -59.675) centre (120.8, -60.175) ccw
  arc A211 (269.725, -40.625) -> (269.225, -41.125) centre (269.725, -41.125) ccw
  line L220 (88.25, -60.175) -> (88.25, -73.175)
  arc A212 (57.7938, -59.675) -> (57.2938, -60.175) centre (57.7938, -60.175) ccw
  arc A213 (316.1193, -41.625) -> (315.6193, -42.125) centre (316.1193, -42.125) ccw
  line L221 (316.1193, -56.625) -> (322.1193, -56.625)
  line L222 (71.2938, -60.175) -> (71.2938, -73.175)
  line L223 (292.2432, -41.625) -> (298.2432, -41.625)
  arc A214 (49.3558, -60.675) -> (48.8558, -61.175) centre (49.3558, -61.175) ccw
  arc A215 (174.475, -40.625) -> (173.975, -41.125) centre (174.475, -41.125) ccw
  line L224 (322.6192, -42.125) -> (322.6193, -56.125)
  arc A216 (315.6193, -56.125) -> (316.1193, -56.625) centre (316.1193, -56.125) ccw
  arc A217 (322.1193, -56.625) -> (322.6193, -56.125) centre (322.1193, -56.125) ccw
  line L225 (73.2318, -60.675) -> (79.2318, -60.675)
  arc A218 (79.2318, -75.675) -> (79.7318, -75.175) centre (79.2318, -75.175) ccw
  line L226 (88.75, -59.675) -> (101.75, -59.675)
  line L227 (48.8558, -61.175) -> (48.8558, -75.175)
  arc A219 (298.7432, -42.125) -> (298.2432, -41.625) centre (298.2432, -42.125) ccw
  line L228 (88.75, -73.675) -> (101.75, -73.675)
  arc A220 (88.75, -59.675) -> (88.25, -60.175) centre (88.75, -60.175) ccw
  arc A221 (298.2432, -56.625) -> (298.7432, -56.125) centre (298.2432, -56.125) ccw
  line L229 (72.7318, -61.175) -> (72.7318, -75.175)
  arc A222 (79.7318, -61.175) -> (79.2318, -60.675) centre (79.2318, -61.175) ccw
  arc A223 (300.6812, -40.625) -> (300.1812, -41.125) centre (300.6812, -41.125) ccw
  line L230 (291.7432, -42.125) -> (291.7432, -56.125)
  line L231 (49.3558, -60.675) -> (55.3558, -60.675)
  arc A224 (88.25, -73.175) -> (88.75, -73.675) centre (88.75, -73.175) ccw
  arc A225 (101.75, -73.675) -> (102.25, -73.175) centre (101.75, -73.175) ccw
  arc A226 (55.3558, -75.675) -> (55.8558, -75.175) centre (55.3558, -75.175) ccw
  arc A227 (235.6, -60.175) -> (235.1, -59.675) centre (235.1, -60.175) ccw
  line L232 (159.4, -60.175) -> (159.4, -73.175)
  line L233 (107.3, -60.175) -> (107.3, -73.175)
  arc A228 (145.9, -59.675) -> (145.4, -60.175) centre (145.9, -60.175) ccw
  arc A229 (241.15, -59.675) -> (240.65, -60.175) centre (241.15, -60.175) ccw
  line L234 (273.7, -60.175) -> (273.7, -73.175)
  arc A230 (140.35, -60.175) -> (139.85, -59.675) centre (139.85, -60.175) ccw
  line L235 (203.05, -73.675) -> (216.05, -73.675)
  line L236 (107.8, -59.675) -> (120.8, -59.675)
  line L237 (178.45, -60.175) -> (178.45, -73.175)
  line L238 (241.15, -73.675) -> (254.15, -73.675)
  arc A231 (126.35, -73.175) -> (126.85, -73.675) centre (126.85, -73.175) ccw
  line L239 (164.95, -59.675) -> (177.95, -59.675)
  arc A232 (222.1, -59.675) -> (221.6, -60.175) centre (222.1, -60.175) ccw
  line L240 (145.9, -73.675) -> (158.9, -73.675)
  arc A233 (139.85, -73.675) -> (140.35, -73.175) centre (139.85, -73.175) ccw
  arc A234 (164.95, -59.675) -> (164.45, -60.175) centre (164.95, -60.175) ccw
  arc A235 (254.65, -60.175) -> (254.15, -59.675) centre (254.15, -60.175) ccw
  line L241 (216.55, -60.175) -> (216.55, -73.175)
  line L242 (183.5, -60.175) -> (183.5, -73.175)
  line L243 (235.6, -60.175) -> (235.6, -73.175)
  line L244 (295.9188, -59.675) -> (308.9188, -59.675)
  arc A236 (203.05, -59.675) -> (202.55, -60.175) centre (203.05, -60.175) ccw
  line L245 (222.1, -59.675) -> (235.1, -59.675)
  arc A237 (202.55, -73.175) -> (203.05, -73.675) centre (203.05, -73.175) ccw
  line L246 (164.95, -73.675) -> (177.95, -73.675)
  arc A238 (216.05, -73.675) -> (216.55, -73.175) centre (216.05, -73.175) ccw
  arc A239 (259.7, -73.175) -> (260.2, -73.675) centre (260.2, -73.175) ccw
  line L247 (309.4187, -60.175) -> (309.4187, -73.175)
  arc A240 (159.4, -60.175) -> (158.9, -59.675) centre (158.9, -60.175) ccw
  arc A241 (221.6, -73.175) -> (222.1, -73.675) centre (222.1, -73.175) ccw
  line L248 (184, -73.675) -> (197, -73.675)
  arc A242 (197, -73.675) -> (197.5, -73.175) centre (197, -73.175) ccw
  arc A243 (273.2, -73.675) -> (273.7, -73.175) centre (273.2, -73.175) ccw
  arc A244 (145.4, -73.175) -> (145.9, -73.675) centre (145.9, -73.175) ccw
  line L249 (260.2, -59.675) -> (273.2, -59.675)
  arc A245 (260.2, -59.675) -> (259.7, -60.175) centre (260.2, -60.175) ccw
  arc A246 (254.15, -73.675) -> (254.65, -73.175) centre (254.15, -73.175) ccw
  arc A247 (164.45, -73.175) -> (164.95, -73.675) centre (164.95, -73.175) ccw
  line L250 (197.5, -60.175) -> (197.5, -73.175)
  arc A248 (183.5, -73.175) -> (184, -73.675) centre (184, -73.175) ccw
  line L251 (240.65, -60.175) -> (240.65, -73.175)
  line L252 (260.2, -73.675) -> (273.2, -73.675)
  arc A249 (235.1, -73.675) -> (235.6, -73.175) centre (235.1, -73.175) ccw
  arc A250 (158.9, -73.675) -> (159.4, -73.175) centre (158.9, -73.175) ccw
  line L253 (184, -59.675) -> (197, -59.675)
  arc A251 (184, -59.675) -> (183.5, -60.175) centre (184, -60.175) ccw
  line L254 (203.05, -59.675) -> (216.05, -59.675)
  line L255 (254.65, -60.175) -> (254.65, -73.175)
  line L256 (202.55, -60.175) -> (202.55, -73.175)
  arc A252 (240.65, -73.175) -> (241.15, -73.675) centre (241.15, -73.175) ccw
  arc A253 (273.7, -60.175) -> (273.2, -59.675) centre (273.2, -60.175) ccw
  arc A254 (178.45, -60.175) -> (177.95, -59.675) centre (177.95, -60.175) ccw
  line L257 (326.0875, -60.175) -> (326.0875, -73.175)
  line L258 (241.15, -59.675) -> (254.15, -59.675)
  line L259 (311.3567, -60.675) -> (311.5875, -60.675)
  line L260 (295.9188, -73.675) -> (308.9188, -73.675)
  arc A255 (197.5, -60.175) -> (197, -59.675) centre (197, -60.175) ccw
  arc A256 (354.6625, -60.175) -> (354.1625, -59.675) centre (354.1625, -60.175) ccw
  arc A257 (177.95, -73.675) -> (178.45, -73.175) centre (177.95, -73.175) ccw
  line L261 (340.6625, -60.175) -> (340.6625, -73.175)
  line L262 (285.8937, -60.175) -> (285.8937, -73.175)
  arc A258 (71.5812, -92.225) -> (72.0812, -92.725) centre (72.0812, -92.225) ccw
  arc A259 (126.85, -59.675) -> (126.35, -60.175) centre (126.85, -60.175) ccw
  line L263 (221.6, -60.175) -> (221.6, -73.175)
  line L264 (164.45, -60.175) -> (164.45, -73.175)
  line L265 (259.7, -60.175) -> (259.7, -73.175)
  line L266 (312.0875, -60.175) -> (312.0875, -60.175)
  arc A260 (85.5813, -79.225) -> (85.0812, -78.725) centre (85.0812, -79.225) ccw
  line L267 (48.2688, -78.725) -> (61.2688, -78.725)
  line L268 (293.9808, -74.175) -> (293.9808, -75.175)
  arc A261 (293.4808, -75.675) -> (293.9808, -75.175) centre (293.4808, -75.175) ccw
  line L269 (341.1625, -59.675) -> (354.1625, -59.675)
  arc A262 (354.1625, -73.675) -> (354.6625, -73.175) centre (354.1625, -73.175) ccw
  line L270 (287.4808, -75.675) -> (293.4808, -75.675)
  line L271 (145.4, -60.175) -> (145.4, -73.175)
  line L272 (145.9, -59.675) -> (158.9, -59.675)
  line L273 (85.5813, -79.225) -> (85.5813, -92.225)
  line L274 (95.8938, -92.725) -> (108.8938, -92.725)
  line L275 (286.3937, -59.675) -> (299.3938, -59.675)
  arc A263 (317.3568, -75.675) -> (317.8568, -75.175) centre (317.3568, -75.175) ccw
  line L276 (222.1, -73.675) -> (235.1, -73.675)
  arc A264 (216.55, -60.175) -> (216.05, -59.675) centre (216.05, -60.175) ccw
  arc A265 (310.8567, -75.175) -> (311.3567, -75.675) centre (311.3567, -75.175) ccw
  arc A266 (309.4187, -60.175) -> (308.9187, -59.675) centre (308.9187, -60.175) ccw
  line L277 (341.1625, -73.675) -> (354.1625, -73.675)
  arc A267 (341.1625, -59.675) -> (340.6625, -60.175) centre (341.1625, -60.175) ccw
  line L278 (317.8568, -74.175) -> (317.8568, -75.175)
  arc A268 (311.3567, -60.675) -> (310.8567, -61.175) centre (311.3567, -61.175) ccw
  line L279 (109.3937, -79.225) -> (109.3937, -92.225)
  line L280 (72.0812, -92.725) -> (85.0812, -92.725)
  line L281 (48.2688, -92.725) -> (61.2688, -92.725)
  arc A269 (47.7688, -92.225) -> (48.2688, -92.725) centre (48.2688, -92.225) ccw
  line L282 (312.5875, -59.675) -> (325.5875, -59.675)
  arc A270 (340.6625, -73.175) -> (341.1625, -73.675) centre (341.1625, -73.175) ccw
  arc A271 (286.3937, -59.675) -> (285.8937, -60.175) centre (286.3937, -60.175) ccw
  line L283 (95.3937, -79.225) -> (95.3937, -92.225)
  line L284 (47.7687, -79.225) -> (47.7688, -92.225)
  arc A272 (326.0875, -60.175) -> (325.5875, -59.675) centre (325.5875, -60.175) ccw
  arc A273 (308.9187, -73.675) -> (309.4187, -73.175) centre (308.9187, -73.175) ccw
  line L285 (61.7687, -79.225) -> (61.7687, -92.225)
  line L286 (286.9808, -74.175) -> (286.9808, -75.175)
  line L287 (354.6625, -60.175) -> (354.6625, -73.175)
  line L288 (71.5812, -79.225) -> (71.5812, -92.225)
  arc A274 (312.5875, -59.675) -> (312.0875, -60.175) centre (312.5875, -60.175) ccw
  arc A275 (286.9808, -75.175) -> (287.4808, -75.675) centre (287.4808, -75.175) ccw
  arc A276 (109.3938, -79.225) -> (108.8938, -78.725) centre (108.8938, -79.225) ccw
  line L289 (310.8567, -61.175) -> (310.8567, -75.175)
  arc A277 (238.7688, -78.725) -> (238.2688, -79.225) centre (238.7688, -79.225) ccw
  arc A278 (227.3313, -80.225) -> (226.8313, -79.725) centre (226.8313, -80.225) ccw
  arc A279 (226.8313, -94.725) -> (227.3313, -94.225) centre (226.8313, -94.225) ccw
  arc A280 (238.2688, -92.225) -> (238.7688, -92.725) centre (238.7688, -92.225) ccw
  arc A281 (251.7687, -92.725) -> (252.2687, -92.225) centre (251.7687, -92.225) ccw
  line L290 (262.5813, -78.725) -> (275.5813, -78.725)
  arc A282 (72.0812, -78.725) -> (71.5812, -79.225) centre (72.0812, -79.225) ccw
  line L291 (180.8313, -79.225) -> (180.8313, -92.225)
  arc A283 (262.5813, -78.725) -> (262.0813, -79.225) centre (262.5813, -79.225) ccw
  line L292 (318.3568, -73.675) -> (325.5875, -73.675)
  arc A284 (180.8313, -79.225) -> (180.3313, -78.725) centre (180.3313, -79.225) ccw
  arc A285 (325.5875, -73.675) -> (326.0875, -73.175) centre (325.5875, -73.175) ccw
  line L293 (95.8938, -78.725) -> (108.8938, -78.725)
  line L294 (72.0812, -78.725) -> (85.0812, -78.725)
  line L295 (311.3567, -75.675) -> (317.3567, -75.675)
  arc A286 (61.7687, -79.225) -> (61.2687, -78.725) centre (61.2687, -79.225) ccw
  arc A287 (85.0812, -92.725) -> (85.5813, -92.225) centre (85.0812, -92.225) ccw
  line L296 (166.8313, -79.225) -> (166.8313, -92.225)
  arc A288 (180.3313, -92.725) -> (180.8313, -92.225) centre (180.3313, -92.225) ccw
  arc A289 (220.3313, -94.225) -> (220.8313, -94.725) centre (220.8313, -94.225) ccw
  line L297 (238.2688, -79.225) -> (238.2688, -92.225)
  arc A290 (285.8937, -73.175) -> (286.3937, -73.675) centre (286.3937, -73.175) ccw
  arc A291 (61.2687, -92.725) -> (61.7688, -92.225) centre (61.2687, -92.225) ccw
  arc A292 (48.2688, -78.725) -> (47.7688, -79.225) centre (48.2688, -79.225) ccw
  arc A293 (220.8313, -79.725) -> (220.3313, -80.225) centre (220.8313, -80.225) ccw
  line L298 (167.3313, -78.725) -> (180.3313, -78.725)
  arc A294 (108.8938, -92.725) -> (109.3938, -92.225) centre (108.8938, -92.225) ccw
  line L299 (127.3313, -80.225) -> (127.3313, -94.225)
  line L300 (252.2688, -79.225) -> (252.2688, -92.225)
  line L301 (220.8313, -94.725) -> (226.8313, -94.725)
  arc A295 (95.8938, -78.725) -> (95.3938, -79.225) centre (95.8938, -79.225) ccw
  line L302 (120.8313, -79.725) -> (126.8313, -79.725)
  arc A296 (120.8313, -79.725) -> (120.3313, -80.225) centre (120.8313, -80.225) ccw
  arc A297 (167.3313, -78.725) -> (166.8313, -79.225) centre (167.3313, -79.225) ccw
  arc A298 (166.8313, -92.225) -> (167.3313, -92.725) centre (167.3313, -92.225) ccw
  line L303 (120.8313, -94.725) -> (126.8313, -94.725)
  arc A299 (127.3313, -80.225) -> (126.8313, -79.725) centre (126.8313, -80.225) ccw
  line L304 (120.3312, -80.225) -> (120.3312, -94.225)
  line L305 (227.3313, -80.225) -> (227.3313, -94.225)
  line L306 (238.7688, -78.725) -> (251.7687, -78.725)
  line L307 (262.0813, -79.225) -> (262.0813, -92.225)
  line L308 (220.8313, -79.725) -> (226.8313, -79.725)
  arc A300 (126.8313, -94.725) -> (127.3313, -94.225) centre (126.8313, -94.225) ccw
  arc A301 (120.3313, -94.225) -> (120.8313, -94.725) centre (120.8313, -94.225) ccw
  line L309 (167.3313, -92.725) -> (180.3313, -92.725)
  arc A302 (95.3938, -92.225) -> (95.8938, -92.725) centre (95.8938, -92.225) ccw
  line L310 (220.3313, -80.225) -> (220.3313, -94.225)
  line L311 (262.5813, -92.725) -> (275.5813, -92.725)
  line L312 (238.7688, -92.725) -> (251.7687, -92.725)
  line L313 (276.0813, -79.225) -> (276.0813, -92.225)
  arc A303 (252.2687, -79.225) -> (251.7687, -78.725) centre (251.7687, -79.225) ccw
  line L314 (268.9375, -9.525) -> (273.9875, -9.525)
  arc A304 (293.5375, -2.525) -> (293.0375, -3.025) centre (293.5375, -3.025) ccw
  line L315 (312.5875, -2.525) -> (325.5875, -2.525)
  arc A305 (293.0375, -16.025) -> (293.5375, -16.525) centre (293.5375, -16.025) ccw
  line L316 (293.5375, -2.525) -> (306.5375, -2.525)
  arc A306 (325.5875, -16.525) -> (326.0875, -16.025) centre (325.5875, -16.025) ccw
  line L317 (326.0875, -3.025) -> (326.0875, -16.025)
  line L318 (293.0375, -3.025) -> (293.0375, -16.025)
  arc A307 (326.0875, -3.025) -> (325.5875, -2.525) centre (325.5875, -3.025) ccw
  line L319 (293.5375, -16.525) -> (293.6245, -16.525)
  line L320 (301.6245, -16.525) -> (306.5375, -16.525)
  line L321 (312.5875, -16.525) -> (317.5005, -16.525)
  line L322 (325.5005, -16.525) -> (325.5875, -16.525)
  arc A308 (301.6245, -16.525) -> (301.1245, -17.025) centre (301.6245, -17.025) ccw
  arc A309 (294.1245, -17.025) -> (293.6245, -16.525) centre (293.6245, -17.025) ccw
  arc A310 (318.0005, -17.025) -> (317.5005, -16.525) centre (317.5005, -17.025) ccw
  arc A311 (325.5005, -16.525) -> (325.0005, -17.025) centre (325.5005, -17.025) ccw
  line L323 (286.3937, -73.675) -> (286.4808, -73.675)
  line L324 (294.4808, -73.675) -> (299.3938, -73.675)
  arc A312 (311.5875, -60.675) -> (312.0875, -60.175) centre (311.5875, -60.175) ccw
  arc A313 (294.4808, -73.675) -> (293.9808, -74.175) centre (294.4808, -74.175) ccw
  arc A314 (286.9808, -74.175) -> (286.4808, -73.675) centre (286.4808, -74.175) ccw
  arc A315 (318.3568, -73.675) -> (317.8568, -74.175) centre (318.3568, -74.175) ccw
  line L325 (40.3875, 2.475) -> (475.8604, 2.475)
  line L326 (475.8604, 2.475) -> (475.8604, -97.725)
  line L327 (40.3875, -97.725) -> (40.3875, 2.475)
  line L328 (54.7687, -92.725) -> (54.7687, -97.725)
  line L329 (40.3875, -97.725) -> (475.8604, -97.725)
  line L330 (383.7929, -34.7152) -> (459.7929, -34.7152)
  line L331 (459.7929, -88.7152) -> (383.7929, -88.7152)
  line L332 (459.7929, -44.7152) -> (463.5139, -44.7152)
  arc A316 (463.5139, -48.8568) -> (463.5139, -44.7152) centre (463.5139, -46.786) ccw
  line L333 (463.5139, -48.8568) -> (459.7929, -48.8568)
  line L334 (383.7929, -44.7152) -> (380.072, -44.7152)
  arc A317 (380.072, -44.7152) -> (380.072, -48.8568) centre (380.072, -46.786) ccw
  line L335 (380.072, -48.8568) -> (383.7929, -48.8568)
  circle A318 centre (463.5139, -46.786) radius 1
  line L336 (383.7929, -88.7152) -> (383.7929, -48.8568)
  line L337 (383.7929, -44.7152) -> (383.7929, -34.7152)
  circle A319 centre (380.072, -46.786) radius 1
  line L338 (459.7929, -34.7152) -> (459.7929, -44.7152)
  line L339 (459.7929, -48.8568) -> (459.7929, -88.7152)
  dimension "d1" = 5.05
  dimension "d3" = 5.05
  dimension "d4" = 0.5
  dimension "d5" = 0.5
  dimension "d6" = 0.5
  dimension "d7" = 0.5
  dimension "d9" = 0.5
  dimension "d10" = 0.5
  dimension "d11" = 0.5
  dimension "d12" = 0.5
  dimension "d13" = 5
  dimension "d14" = 5
  dimension "d17" = 5
  dimension "d18" = 76
  dimension "d19" = 54
  dimension "d20" = 2
  dimension "d21" = 2
  dimension "d39" = 10
  constraint midpoint L56 L314.start
  constraint midpoint L51 L314.end
  constraint collinear L319 L320
  constraint collinear L321 L322
  constraint tangent L47 A308
  constraint tangent L320 A308
  constraint tangent L319 A309
  constraint tangent L41 A309
  constraint tangent L95 A310
  constraint tangent L321 A310
  constraint tangent L322 A311
  constraint tangent L82 A311
  constraint collinear L257 L317
  constraint collinear L323 L324
  constraint tangent L259 A312
  constraint tangent L268 A313
  constraint tangent L324 A313
  constraint tangent L286 A314
  constraint tangent L323 A314
  constraint tangent L278 A315
  constraint tangent L292 A315
  constraint collinear L29 L176
  constraint horizontal L325
  constraint vertical L326
  constraint vertical L327
  constraint midpoint L281 L328.start
  constraint perpendicular L281 L328
  constraint perpendicular L326 L329
  constraint horizontal L330
  constraint vertical L338
  constraint horizontal L331
  constraint vertical L336
  constraint perpendicular L332 L338
  constraint tangent L332 A316
  constraint coincident L333.end L338
  constraint tangent A316 L333
  constraint perpendicular L333 L338
  constraint coincident L334.start L336
  constraint perpendicular L334 L336
  constraint tangent L334 A317
  constraint tangent A317 L335
  constraint perpendicular L335 L336
  constraint collinear L333 L335
  constraint collinear L332 L334
  constraint equal L332 L334
  constraint concentric A316 A318
  constraint collinear L336 L337
  constraint concentric A317 A319
  constraint collinear L338 L339
  measures "d1" distance of L314.start L314.end
  measures "d3" distance of L71 L318
  measures "d4" radius of A308
  measures "d5" radius of A309
  measures "d6" radius of A310
  measures "d7" radius of A311
  measures "d9" radius of A312
  measures "d10" radius of A313
  measures "d11" radius of A314
  measures "d12" radius of A315
  measures "d13" distance of L50 L325
  measures "d14" distance of L29 L327
  measures "d17" distance of L328.start L328.end
  measures "d18" distance of L330.start L330.end
  measures "d19" distance of L330.end L331.start
  measures "d20" diameter of A318
  measures "d21" diameter of A319
  measures "d39" distance of L330.start L334.start
mesh "Mesh1" [no effect]
extrude "Extrude1" add sketch "plate-20210524-013526" along normal blind 3 contours L325 L326 L327 L329 makes body 1 in component "Plate"